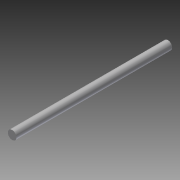
# Autodesk Inventor part: Shaft (0.500 Aluminum
Saved by Autodesk Inventor 2014 (Build 180170000, 170)
## iProperties
Created: 2014-01-12
Part Number: Shaft (0.500 Aluminum
Material: Steel
Document SubType Name: Modeling
Designer: Andrew Toennies
Mass: 227.323 g
Surface Area: 93.7409 cm^2
Volume: 28.9583 cm^3
Density: 7.85 g/cm^3
Appearance: Steel
Author: Andrew Toennies
Autodesk Inventor part; units mm, degrees
ref_plane "YZ Plane" through (0, 0, 0) normal (1, 0, 0) x (0, 1, 0)
ref_plane "XZ Plane" through (0, 0, 0) normal (0, 1, 0) x (-1, 0, 0)
ref_plane "XY Plane" through (0, 0, 0) normal (0, 0, 1) x (1, 0, 0)
sketch "Sketch1" plane through (0, 0, 0) normal (0, 0, 1) x (1, 0, 0)
  circle A0 centre (0, 0) radius 6.35
  circle A1 centre (0, 0) radius 5.6388
  dimension "d0" = 12.7
  dimension "d3" = 0.7112
  constraints: 2 centre point, 1 coincident
  measures "d0" diameter of A0
  measures "d3" radial gap between concentric circles of A0 A1
extrude "Extrusion1" add sketch "Sketch1" along normal blind 177.8
body "Solid1"
